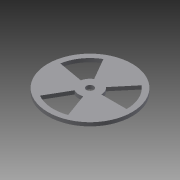
# Autodesk Inventor part: main_wheel
Saved by Autodesk Inventor 2014 SP2 (Build 180246200, 246)
## iProperties
Created: 2015-11-29
Part Number: main_wheel
Material: Generic
Document SubType Name: Modeling
Designer: schrluka
Density: 1 g/cm^3
Appearance: Default
Author: schrluka
Autodesk Inventor part; units mm, degrees
ref_plane "YZ Plane" through (0, 0, 0) normal (1, 0, 0) x (0, 1, 0)
ref_plane "XZ Plane" through (0, 0, 0) normal (0, 1, 0) x (-1, 0, 0)
ref_plane "XY Plane" through (0, 0, 0) normal (0, 0, 1) x (1, 0, 0)
sketch "Sketch1" plane through (0, 0, 0) normal (0, 0, 1) x (1, 0, 0)
  circle A0 centre (0, 0) radius 46.5 projected
extrude "Extrusion1" add sketch "Sketch1" along normal mid plane 6
sketch "Sketch2" plane through (0, 0, 3) normal (0, 0, 1) x (1, 0, 0)
  circle A0 centre (0, 0) radius 46.5 projected
  circle A1 centre (0, 0) radius 4.5 projected
  arc A2 (17.272, -47.4545) -> (50.5, 0) centre (0, 0) ccw projected
  line L0 (17.272, -47.4545) -> (4.2753, -11.7462) projected
  arc A3 (-6.25, -10.8253) -> (4.2753, -11.7462) centre (0, 0) ccw projected
  line L1 (-6.25, -10.8253) -> (-25.25, -43.7343) projected
  arc A4 (-49.7328, 8.7692) -> (-25.25, -43.7343) centre (0, 0) ccw projected
  line L2 (-49.7328, 8.7692) -> (-12.3101, 2.1706) projected
  arc A5 (-6.25, 10.8253) -> (-12.3101, 2.1706) centre (0, 0) ccw projected
  line L3 (-6.25, 10.8253) -> (-25.25, 43.7343) projected
  arc A6 (32.4608, 38.6852) -> (-25.25, 43.7343) centre (0, 0) ccw projected
  line L4 (32.4608, 38.6852) -> (8.0348, 9.5756) projected
  arc A7 (12.5, 0) -> (8.0348, 9.5756) centre (0, 0) ccw projected
  line L5 (12.5, 0) -> (50.5, 0) projected
  circle A8 centre (0, 0) radius 40.5 construction
  arc A9 (40.5, 0) -> (26.0329, 31.0248) centre (0, 0) ccw
  arc A10 (-20.25, 35.074) -> (-39.8847, 7.0328) centre (0, 0) ccw
  arc A11 (-20.25, -35.074) -> (13.8518, -38.0576) centre (0, 0) ccw
  point P0 (-23.25, -40.2702)
  point P1 (15.9039, -43.6957)
  point P2 (-23.25, 40.2702)
  point P3 (-45.7936, 8.0746)
  point P4 (46.5, 0)
  point P5 (29.8896, 35.6211)
  dimension "d4" = 6
  constraints: 12 point on circle, 12 point on line, 4 centre point, 3 coincident
  measures "d4" radial gap between concentric circles of A0 A8
extrude "Extrusion3" cut sketch "Sketch2" against normal through all contours L5 A7 L4 A9 | A11 L1 A3 L0 | L3 A5 L2 A10
sketch "Sketch3" plane through (0, 0, 3) normal (0, 0, 1) x (1, 0, 0)
  circle A0 centre (0, 0) radius 46.5 projected
  constraints: 1 coincident
hole "Hole1" at (0, 0, 3) direction (0, 0, -1) diameter 8 end through all
body "Solid1"
